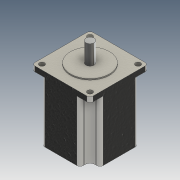
# Autodesk Inventor part: nema23-wotiom
Saved by Autodesk Inventor 2017 (Build 210142000, 142)
## iProperties
Created: 2018-05-10
Part Number: nema23-wotiom
Material: Generic
Document SubType Name: Modeling
Designer: Luiz Gustavo
Density: 1 g/cm^3
Appearance: Default
Author: Luiz Gustavo
Autodesk Inventor part; units mm, degrees
ref_plane "YZ Plane" through (0, 0, 0) normal (1, 0, 0) x (0, 1, 0)
ref_plane "XZ Plane" through (0, 0, 0) normal (0, 1, 0) x (-1, 0, 0)
ref_plane "XY Plane" through (0, 0, 0) normal (0, 0, 1) x (1, 0, 0)
sketch "Sketch1" plane through (0, 0, 0) normal (0, 0, 1) x (1, 0, 0)
  line L0 (-28.5, -28.5) -> (28.5, -28.5)
  line L1 (28.5, -28.5) -> (28.5, 28.5)
  line L2 (28.5, 28.5) -> (-28.5, 28.5)
  line L3 (-28.5, 28.5) -> (-28.5, -28.5)
  line L4 (-28.5, -28.5) -> (28.5, 28.5) construction
  line L5 (28.5, -28.5) -> (-28.5, 28.5) construction
  circle A0 centre (23.57, 23.57) radius 2.55
  line L6 (0, 28.5) -> (0, -28.5) construction
  line L7 (28.5, 0) -> (-28.5, 0) construction
  circle A1 centre (-23.57, 23.57) radius 2.55
  circle A2 centre (23.57, -23.57) radius 2.55
  circle A3 centre (-23.57, -23.57) radius 2.55
  circle A4 centre (0, 0) radius 19.05
  circle A5 centre (0, 0) radius 4
  dimension "d0" = 57
  dimension "d1" = 57
  dimension "d2" = 5.1
  dimension "d3" = 47.14
  dimension "d4" = 38.1
  dimension "d5" = 8
  constraints: 16 end point, 6 centre point, 6 midpoint, 3 symmetric about line, 2 coincident, 2 parallel, 1 horizontal, 1 perpendicular, 1 point on line, 3 other
  measures "d0" distance of L2.end L1.end
  measures "d1" distance of L1.end L0.end
  measures "d2" diameter of A0
  measures "d3" distance of A0.centre A1.centre
  measures "d4" diameter of A4
  measures "d5" diameter of A5
extrude "Extrusion1" add sketch "Sketch1" against normal blind 64 contours L3 L2 L1 L0 | A4 | A5
extrude "Extrusion2" add sketch "Sketch1" along normal blind 1.2 contours A4
extrude "Extrusion3" add sketch "Sketch1" along normal blind 20.2 contours A5
sketch "Sketch2" plane through (0, 0, -64) normal (0, 0, -1) x (-1, 0, 0)
  circle A0 centre (-23.57, -23.57) radius 2.55 projected
  circle A1 centre (23.57, -23.57) radius 2.55 projected
  circle A2 centre (23.57, 23.57) radius 2.55 projected
  circle A3 centre (-23.57, 23.57) radius 2.55 projected
  line L0 (-28.5, -28.5) -> (28.5, -28.5) projected
  line L1 (28.5, -28.5) -> (28.5, 28.5) projected
  line L2 (28.5, 28.5) -> (-28.5, 28.5) projected
  line L3 (-28.5, 28.5) -> (-28.5, -28.5) projected
  line L4 (-28.5, -28.5) -> (-28.5, 28.5) projected
  line L5 (28.5, 28.5) -> (28.5, -28.5) projected
  line L6 (-18.64, -18.64) -> (-23.57, -18.64) construction
  line L7 (-28.5, -18.64) -> (-28.5, -28.5)
  line L8 (-28.5, -28.5) -> (-18.64, -28.5)
  line L9 (-18.64, -28.5) -> (-18.64, -23.57)
  line L10 (-18.64, -18.64) -> (-28.5, -28.5) construction
  line L11 (-28.5, -18.64) -> (-18.64, -28.5) construction
  line L12 (-28.5, 28.5) -> (28.5, 28.5) projected
  circle A4 centre (-23.57, -23.57) radius 2.55 projected
  arc A5 (-27.056, -20.084) -> (-28.5, -23.57) centre (-23.57, -23.57) ccw construction
  line L13 (-18.64, -23.57) -> (-18.64, -18.64) construction
  line L14 (-23.57, -18.64) -> (-28.5, -18.64)
  arc A6 (-23.57, -18.64) -> (-27.056, -20.084) centre (-23.57, -23.57) ccw construction
  arc A7 (-27.056, -27.056) -> (-20.084, -27.056) centre (-23.57, -23.57) ccw construction
  arc A8 (-20.084, -27.056) -> (-18.64, -23.57) centre (-23.57, -23.57) ccw construction
  arc A9 (-20.084, -20.084) -> (-23.57, -18.64) centre (-23.57, -23.57) ccw
  arc A10 (-18.64, -23.57) -> (-20.084, -20.084) centre (-23.57, -23.57) ccw
  arc A11 (-28.5, -23.57) -> (-27.056, -27.056) centre (-23.57, -23.57) ccw construction
  line L15 (0, 28.5) -> (0, -28.5) construction
  line L16 (-28.5, -28.5) -> (28.5, -28.5) construction
  line L17 (28.5, 0) -> (-28.5, 0) construction
  circle A12 centre (23.57, -23.57) radius 2.55
  line L18 (18.64, -18.64) -> (23.57, -18.64) construction
  line L19 (28.5, -18.64) -> (28.5, -28.5)
  line L20 (28.5, -28.5) -> (18.64, -28.5)
  line L21 (18.64, -28.5) -> (18.64, -23.57)
  line L22 (18.64, -18.64) -> (28.5, -28.5) construction
  line L23 (28.5, -18.64) -> (18.64, -28.5) construction
  circle A13 centre (23.57, -23.57) radius 2.55
  arc A14 (28.5, -23.57) -> (27.056, -20.084) centre (23.57, -23.57) ccw construction
  line L24 (18.64, -23.57) -> (18.64, -18.64) construction
  line L25 (23.57, -18.64) -> (28.5, -18.64)
  arc A15 (27.056, -20.084) -> (23.57, -18.64) centre (23.57, -23.57) ccw construction
  arc A16 (20.084, -27.056) -> (27.056, -27.056) centre (23.57, -23.57) ccw construction
  arc A17 (18.64, -23.57) -> (20.084, -27.056) centre (23.57, -23.57) ccw construction
  arc A18 (23.57, -18.64) -> (20.084, -20.084) centre (23.57, -23.57) ccw
  arc A19 (20.084, -20.084) -> (18.64, -23.57) centre (23.57, -23.57) ccw
  arc A20 (27.056, -27.056) -> (28.5, -23.57) centre (23.57, -23.57) ccw construction
  circle A21 centre (-23.57, 23.57) radius 2.55
  circle A22 centre (23.57, 23.57) radius 2.55
  line L26 (-18.64, 18.64) -> (-23.57, 18.64) construction
  line L27 (-28.5, 18.64) -> (-28.5, 28.5)
  line L28 (-28.5, 28.5) -> (-18.64, 28.5)
  line L29 (-18.64, 28.5) -> (-18.64, 23.57)
  line L30 (-18.64, 18.64) -> (-28.5, 28.5) construction
  line L31 (-28.5, 18.64) -> (-18.64, 28.5) construction
  circle A23 centre (-23.57, 23.57) radius 2.55
  arc A24 (-28.5, 23.57) -> (-27.056, 20.084) centre (-23.57, 23.57) ccw construction
  line L32 (-18.64, 23.57) -> (-18.64, 18.64) construction
  line L33 (-23.57, 18.64) -> (-28.5, 18.64)
  arc A25 (-27.056, 20.084) -> (-23.57, 18.64) centre (-23.57, 23.57) ccw construction
  arc A26 (-20.084, 27.056) -> (-27.056, 27.056) centre (-23.57, 23.57) ccw construction
  arc A27 (-18.64, 23.57) -> (-20.084, 27.056) centre (-23.57, 23.57) ccw construction
  arc A28 (-23.57, 18.64) -> (-20.084, 20.084) centre (-23.57, 23.57) ccw
  arc A29 (-20.084, 20.084) -> (-18.64, 23.57) centre (-23.57, 23.57) ccw
  arc A30 (-27.056, 27.056) -> (-28.5, 23.57) centre (-23.57, 23.57) ccw construction
  line L34 (-28.5, 28.5) -> (28.5, 28.5) construction
  circle A31 centre (23.57, 23.57) radius 2.55
  line L35 (18.64, 23.57) -> (18.64, 18.64) construction
  arc A32 (18.64, 23.57) -> (20.084, 20.084) centre (23.57, 23.57) ccw
  line L36 (18.64, 28.5) -> (18.64, 23.57)
  line L37 (18.64, 18.64) -> (23.57, 18.64) construction
  arc A33 (20.084, 27.056) -> (18.64, 23.57) centre (23.57, 23.57) ccw construction
  arc A34 (20.084, 20.084) -> (23.57, 18.64) centre (23.57, 23.57) ccw
  arc A35 (23.57, 18.64) -> (27.056, 20.084) centre (23.57, 23.57) ccw construction
  line L38 (23.57, 18.64) -> (28.5, 18.64)
  arc A36 (27.056, 20.084) -> (28.5, 23.57) centre (23.57, 23.57) ccw construction
  arc A37 (27.056, 27.056) -> (20.084, 27.056) centre (23.57, 23.57) ccw construction
  arc A38 (28.5, 23.57) -> (27.056, 27.056) centre (23.57, 23.57) ccw construction
  line L39 (28.5, 18.64) -> (28.5, 28.5)
  line L40 (18.64, 18.64) -> (28.5, 28.5) construction
  line L41 (28.5, 18.64) -> (18.64, 28.5) construction
  line L42 (28.5, 28.5) -> (18.64, 28.5)
  circle A39 centre (23.57, 23.57) radius 2.55
  point P0 (0, 0)
  constraints: 70 end point, 68 point on circle, 40 symmetric about line, 35 centre point, 17 point on line, 12 midpoint, 4 coincident, 4 parallel, 2 horizontal, 2 perpendicular, 28 other
extrude "Extrusion4" cut sketch "Sketch2" against normal blind 59 contours L3 L14 A9 A10 L9 L0 | L21 A19 A18 L25 L1 L0 | L3 L2 L29 A29 A28 L33 | L38 A34 A32 L36 L2 L1
fillet "Fillet1" radius 3 12 edges at (28.5, 28.5, -2.5) (-28.5, 28.5, -2.5) (-28.5, -28.5, -2.5) (28.5, -28.5, -2.5) (-18.64, -28.5, -34.5) (-28.5, -18.64, -34.5) (18.64, -28.5, -34.5) (28.5, -18.64, -34.5) (28.5, 18.64, -34.5) (18.64, 28.5, -34.5) (-18.64, 28.5, -34.5) (-28.5, 18.64, -34.5)
body "Solid1"
